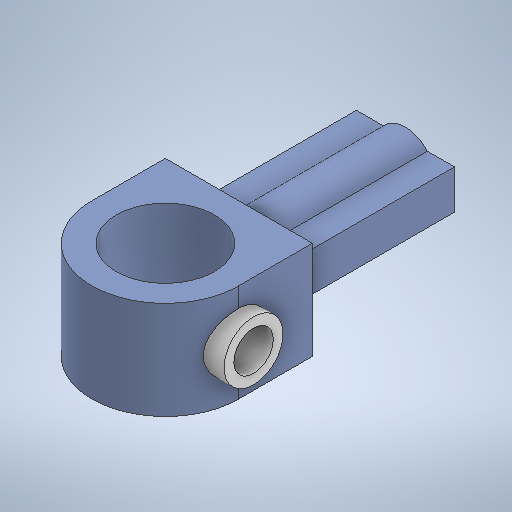
# Autodesk Inventor part: Link_InsideV3
Saved by Autodesk Inventor 2025.1 (Build 291241000, 241)
## iProperties
Created: 2025-01-31
Part Number: Link_InsideV3
Material: Generic
Document SubType Name: Modeling
Designer: m_kni
Density: 1 g/cm^3
Appearance: Default
Author: m_kni
Autodesk Inventor part; units mm, degrees
ref_plane "YZ Plane" through (0, 0, 0) normal (1, 0, 0) x (0, 1, 0)
ref_plane "XZ Plane" through (0, 0, 0) normal (0, 1, 0) x (-1, 0, 0)
ref_plane "XY Plane" through (0, 0, 0) normal (0, 0, 1) x (1, 0, 0)
sketch "Sketch1" plane through (0, 0, 0) normal (0, 1, 0) x (-1, 0, 0)
  line L0 (0, 0) -> (0, -8)
  circle A0 centre (0, -8) radius 3
  line L1 (0, 0) -> (0, 8)
  circle A1 centre (0, 8) radius 2.5
  circle A2 centre (0, 8) radius 3.75
  circle A3 centre (0, -8) radius 3.75
  line L2 (3.75, 8) -> (3.75, -8)
  line L3 (-3.75, 8) -> (-3.75, -8)
  line L4 (3.75, 4.25) -> (-3.75, 4.25)
  line L5 (3.75, -4.25) -> (-3.75, -4.25)
  point P0 (-2.6582, -4.25)
  dimension "d0" = 8
  dimension "d1" = 6
  dimension "d2" = 8
  dimension "d3" = 5
  dimension "d4" = 7.5
  dimension "d5" = 7.5
  dimension "d6" = 8.5
  constraints: 12 end point, 4 centre point, 4 coincident, 4 point on circle, 4 point on line, 4 vertical, 1 horizontal, 1 perpendicular, 1 tangent
  measures "d0" distance of L0.start L0.end
  measures "d1" diameter of A0
  measures "d2" distance of L0.start L1.end
  measures "d3" diameter of A1
  measures "d4" diameter of A2
  measures "d5" diameter of A3
  measures "d6" distance from line of point (-2.658, -4.25) L4
extrude "Extrusion1" add sketch "Sketch1" along normal blind 5 contours L1 L4 L2 L5 L0 | L0 L5 L3 L4 L1 | L4 L3 A2 | A2 | A2 L2 L4
sketch "Sketch2" plane through (3.75, 0, -4.25) normal (0, 0, -1) x (-1, 0, 0)
  line L0 (0, 5) -> (7.5, 5) projected
  line L1 (0, 0) -> (7.5, 0)
  line L2 (7.5, 0) -> (7.5, 5)
  line L3 (7.5, 5) -> (0, 5)
  line L4 (0, 5) -> (0, 0)
  line L5 (0, 0) -> (7.5, 5) construction
  line L6 (7.5, 0) -> (0, 5) construction
  circle A0 centre (3.75, 2.5) radius 1.5
  line L7 (1.25, 1.5) -> (6.25, 1.5)
  line L8 (6.25, 1.5) -> (6.25, 3.5)
  line L9 (6.25, 3.5) -> (1.25, 3.5)
  line L10 (1.25, 3.5) -> (1.25, 1.5)
  line L11 (1.25, 1.5) -> (6.25, 3.5) construction
  line L12 (6.25, 1.5) -> (1.25, 3.5) construction
  point P0 (3.75, 0)
  point P1 (4.868, 1.5)
  point P2 (2.632, 1.5)
  point P3 (2.632, 3.5)
  point P4 (4.868, 3.5)
  dimension "d9" = 3
  dimension "d10" = 5
  dimension "d11" = 2
  constraints: 24 end point, 4 midpoint, 4 parallel, 2 horizontal, 2 perpendicular, 1 centre point, 1 coincident
  measures "d9" diameter of A0
  measures "d10" distance of L9.end L8.end
  measures "d11" distance of L8.end L7.end
extrude "Extrusion2" cut sketch "Sketch2" against normal blind 8.5
sketch "Sketch3" plane through (3.75, 0, 8) normal (1, 0, 0) x (0, 0, -1)
  line L0 (0, 0) -> (0, 5) projected
  circle A0 centre (0, 2.5) radius 1.5
  point P0 (8, 0)
  dimension "d14" = 3
  constraints: 1 centre point, 1 coincident, 1 midpoint
  measures "d14" diameter of A0
extrude "Extrusion3" add sketch "Sketch3" along normal mid plane 1.5
sketch "Sketch4" plane through (4.5, 2.5, 8) normal (1, 0, 0) x (0, 0, -1)
  line L0 (0, -2.5) -> (0, 2.5) projected
  circle A0 centre (0, 0) radius 1
  point P0 (8, -2.5)
  dimension "d17" = 2
  constraints: 1 centre point, 1 midpoint
  measures "d17" diameter of A0
extrude "Extrusion4" cut sketch "Sketch4" against normal blind 3.2625
body "Solid1"
